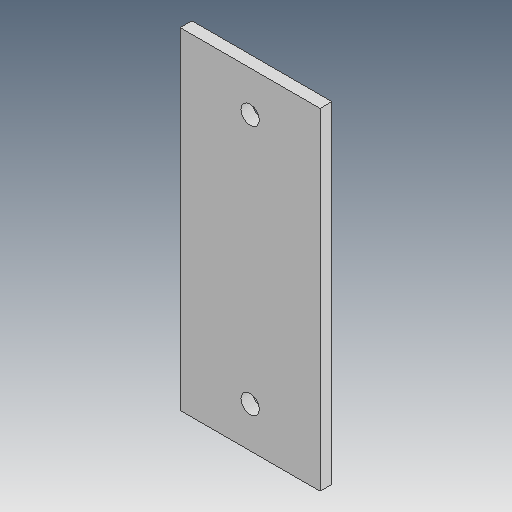
# Autodesk Inventor part: shin_tab
Saved by Autodesk Inventor 2025.2 (Build 292293000, 293)
## iProperties
Created: 2025-02-16
Part Number: shin_tab
Material: Generic
Document SubType Name: Modeling
Designer: email
Density: 1 g/cm^3
Appearance: Default
Author: email
Autodesk Inventor part; units mm, degrees
ref_plane "YZ Plane" through (0, 0, 0) normal (1, 0, 0) x (0, 1, 0)
ref_plane "XZ Plane" through (0, 0, 0) normal (0, 1, 0) x (-1, 0, 0)
ref_plane "XY Plane" through (0, 0, 0) normal (0, 0, 1) x (1, 0, 0)
sketch "Sketch1" plane through (0, 0, 0) normal (0, 0, 1) x (1, 0, 0)
  line L0 (0, 0) -> (38, 0)
  line L1 (38, 0) -> (38, 90)
  line L2 (38, 90) -> (0, 90)
  line L3 (0, 90) -> (0, 0)
  circle A0 centre (19, 79) radius 2.5
  circle A1 centre (19, 11) radius 2.5
  dimension "d0" = 90
  dimension "d1" = 38
  dimension "d2" = 11
  dimension "d3" = 11
  dimension "d4" = 5
  dimension "d5" = 5
  dimension "d6" = 19
  dimension "d9" = 68
  constraints: 8 end point, 2 centre point, 2 parallel, 1 horizontal, 1 perpendicular, 1 vertical alignment
  measures "d0" distance of L0.end L1.end
  measures "d1" distance of L1.end L2.end
  measures "d2" distance from line of L2 A0.centre
  measures "d3" distance from line of L0 A1.centre
  measures "d4" diameter of A0
  measures "d5" diameter of A1
  measures "d6" distance from line of L1 A0.centre
  measures "d9" distance of A1.centre A0.centre
extrude "Extrusion1" add sketch "Sketch1" along normal blind 3.2
body "Solid1"
